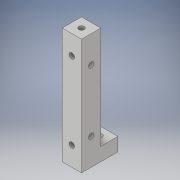
# Autodesk Inventor part: StructureCenter
Saved by Autodesk Inventor 2019 (Build 230136000, 136)
## iProperties
Created: 2020-12-31
Part Number: StructureCenter
Material: Типовые
Document SubType Name: Modeling
Designer: Professional
Density: 1 g/cm^3
Appearance: По умолчанию
Author: Professional
Autodesk Inventor part; units mm, degrees
ref_plane "YZ Plane" through (0, 0, 0) normal (1, 0, 0) x (0, 1, 0)
ref_plane "XZ Plane" through (0, 0, 0) normal (0, 1, 0) x (-1, 0, 0)
ref_plane "XY Plane" through (0, 0, 0) normal (0, 0, 1) x (1, 0, 0)
sketch "Эскиз1" plane through (0, 0, 0) normal (0, 1, 0) x (-1, 0, 0)
  line L0 (0, 0) -> (-10, 0)
  line L1 (-10, 0) -> (-10, -18.8)
  line L2 (-10, -18.8) -> (0, -18.8)
  line L3 (0, -18.8) -> (0, 0)
  point P0 (0, 0)
  dimension "d0" = 10
  dimension "d1" = 18.8
  constraints: 8 end point, 2 parallel, 1 coincident, 1 horizontal, 1 perpendicular
  measures "d0" distance between parallel lines of L1 L3
  measures "d1" distance between parallel lines of L0 L2
extrude "Выдавливание1" add sketch "Эскиз1" along normal blind 7
sketch "Эскиз2" plane through (0, 7, 0) normal (0, 1, 0) x (1, 0, 0)
  line L0 (10, 0) -> (10, 18.8) projected
  line L1 (0, 0) -> (10, 0)
  line L2 (10, 0) -> (10, 10)
  line L3 (10, 10) -> (0, 10)
  line L4 (0, 10) -> (0, 0)
  dimension "d4" = 10
  constraints: 8 end point, 2 parallel, 1 horizontal, 1 perpendicular, 1 point on line
  measures "d4" distance between parallel lines of L1 L3
extrude "Выдавливание2" add sketch "Эскиз2" along normal blind 53
sketch "Эскиз4" plane through (0, 0, 0) normal (0, -1, 0) x (1, 0, 0)
  line L0 (0, 0) -> (10, 0) projected
  line L1 (0, 0) -> (10, 0) projected
  line L2 (10, 0) -> (10, -10) projected
  line L3 (10, -10) -> (0, -10) projected
  line L4 (0, -10) -> (0, 0) projected
  line L5 (0, -10) -> (10, -10) projected
  line L6 (10, -10) -> (10, -18.8) projected
  line L7 (10, -18.8) -> (0, -18.8) projected
  line L8 (0, -18.8) -> (0, -10) projected
  point P0 (5, -5)
  point P1 (5, -14.4)
  point P2 (5, 0)
  point P3 (10, -5)
  point P4 (10, -14.4)
  constraints: 3 midpoint, 2 horizontal alignment, 2 vertical alignment
hole "Отверстие1" at (5, 0, -5) at (5, 0, -14.4) direction (0, 1, 0) diameter 2.8 depth 7
sketch "Эскиз7" plane through (0, 0, 0) normal (0, 0, 1) x (1, 0, 0)
  line L0 (0, 0) -> (10, 0) projected
  line L1 (0, 60) -> (10, 60) projected
  point P0 (5, 10)
  point P1 (5, 50)
  point P2 (5, 0)
  dimension "d21" = 10
  dimension "d22" = 10
  constraints: 2 vertical alignment, 1 midpoint
  measures "d21" distance from line of L0 point (5, 10)
  measures "d22" distance from line of L1 point (5, 50)
hole "Отверстие2" at (5, 10, 0) at (5, 50, 0) direction (0, 0, -1) diameter 2.8 end through all
sketch "Эскиз9" plane through (0, 60, 0) normal (0, 1, 0) x (1, 0, 0)
  circle A0 centre (5, 5) radius 1.4 projected
  point P0 (0, 0)
  constraints: 1 coincident
hole "Отверстие3" at (5, 60, -5) direction (0, -1, 0) diameter 2.8 depth 7
sketch "Эскиз11" plane through (0, 0, -18.8) normal (-1, 0, 0) x (0, 0, 1)
  line L0 (8.8, 60) -> (18.8, 60) projected
  line L1 (0, 0) -> (18.8, 0) projected
  point P0 (13.8, 14)
  point P1 (13.8, 46)
  point P2 (13.8, 60)
  dimension "d37" = 14
  dimension "d38" = 14
  constraints: 2 vertical alignment, 1 midpoint
  measures "d37" distance of point (13.8, 60) point (13.8, 46)
  measures "d38" distance from line of L1 point (13.8, 14)
hole "Отверстие4" at (0, 14, -5) at (0, 46, -5) direction (1, 0, 0) diameter 2.8 end through all
